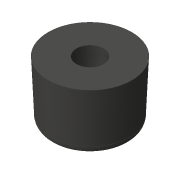
# Autodesk Inventor part: roundBumper
Saved by Autodesk Inventor 2016 SP2 (Build 200236200, 236)
## iProperties
Created: 2017-01-04
Part Number: roundBumper
Material: Rubber
Document SubType Name: Modeling
Designer: sawaiz
Density: 0.93 g/cm^3
Appearance: Rubber - Black
Author: sawaiz
Title: 9540k717
Autodesk Inventor part; units mm, degrees
ref_plane "YZ Plane" through (0, 0, 0) normal (1, 0, 0) x (0, 1, 0)
ref_plane "XZ Plane" through (0, 0, 0) normal (0, 1, 0) x (-1, 0, 0)
ref_plane "XY Plane" through (0, 0, 0) normal (0, 0, 1) x (1, 0, 0)
sketch "Sketch1" plane through (0, 0, 0) normal (0, 1, 0) x (-1, 0, 0)
  circle A0 centre (0, 0) radius 7.9375
  dimension "d0" = 15.875
  constraints: 1 centre point, 1 coincident
  measures "d0" diameter of A0
extrude "Extrusion1" add sketch "Sketch1" along normal blind 11.1125
sketch "Sketch2" plane through (0, 0, 0) normal (0, -1, 0) x (1, 0, 0)
  point P0 (0, 0)
  point P1 (0, 0)
  constraints: 1 coincident
hole "Hole1" at (0, 0, 0) direction (0, 1, 0) diameter 5.1594 end through all counterbore diameter 7.9375 counterbore depth 6.35
draft "FaceDraft1" angle 2.5 pull direction (0, -1, 0) faces at (-7.8347, 7.4083, -1.2733) fixed edges at (7.9375, 11.1125, 0)
fillet "Fillet1" radius 1.5875 1 edges at (7.4523, 0, 0)
body "Solid1"
